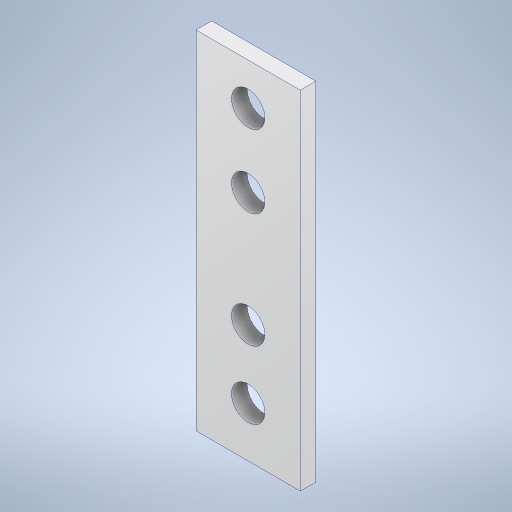
# Autodesk Inventor part: wheel_setter_plate
Saved by Autodesk Inventor 2024.1 (Build 281209000, 209)
## iProperties
Created: 2025-02-03
Part Number: wheel_setter_plate
Material: アルミニウム 6061
Document SubType Name: Sheet Metal
Designer: hibik
Density: 2.7 g/cm^3
Sheet Metal Rule: Default_mm
Appearance: アルミニウム - フラット
Author: hibik
Autodesk Inventor part; units mm, degrees
ref_plane "YZ Plane" through (0, 0, 0) normal (1, 0, 0) x (0, 1, 0)
ref_plane "XZ Plane" through (0, 0, 0) normal (0, 1, 0) x (-1, 0, 0)
ref_plane "XY Plane" through (0, 0, 0) normal (0, 0, 1) x (1, 0, 0)
sketch "スケッチ1" plane through (0, 0, 0) normal (0, 0, 1) x (1, 0, 0)
  line L0 (0, 0) -> (10, 0)
  line L1 (10, 0) -> (10, 35)
  line L2 (10, 35) -> (0, 35)
  line L3 (0, 35) -> (0, 0)
  circle A0 centre (5, 31) radius 1.6
  circle A1 centre (5, 24) radius 1.6
  line L4 (0, 18) -> (10, 18)
  circle A2 centre (5, 13) radius 1.6
  circle A3 centre (5, 6.5) radius 1.6
  line L5 (0, 20) -> (10, 20)
  line L6 (0, 27.5) -> (10, 27.5)
  line L7 (0, 0) -> (10, 0)
  line L8 (10, 0) -> (10, 1.7632)
  line L9 (0, 1.7632) -> (0, 0)
  point P0 (5, 35)
  dimension "d0" = 10
  dimension "d1" = 35
  dimension "d3" = 3.2
  dimension "d4" = 3.2
  dimension "d6" = 7
  dimension "d7" = 18
  dimension "d8" = 3.2
  dimension "d9" = 3.2
  dimension "d10" = 6.5
  dimension "d11" = 5
  dimension "d12" = 15
  measures "d0" distance of L2.end L1.end
  measures "d1" distance of L1.end L0.end
  measures "d3" diameter of A0
  measures "d4" diameter of A1
  measures "d6" distance of A1.centre A0.centre
  measures "d7" distance between parallel lines of L0 L4
  measures "d8" diameter of A2
  measures "d9" diameter of A3
  measures "d10" distance from line of L0 A3.centre
  measures "d11" distance from line of L4 A2.centre
  measures "d12" distance between parallel lines of L2 L5
extrude "プレート1" add sketch "スケッチ1" along normal blind 1.5
sketch "スケッチ2" plane through (0, 0, 1.5) normal (0, 0, 1) x (1, 0, 0)
  line L0 (0, 35) -> (0, 0) projected
  line L1 (10, 0) -> (10, 35) projected
  line L2 (0, 0) -> (10, 0)
  line L3 (10, 0) -> (10, 1.7)
  line L4 (10, 1.7) -> (0, 1.7)
  line L5 (0, 1.7) -> (0, 0)
  dimension "d14" = 1.7
  constraints: 8 end point, 2 parallel, 1 horizontal, 1 perpendicular, 1 point on line
  measures "d14" distance between parallel lines of L2 L4
extrude "切り取り1" cut sketch "スケッチ2" against normal blind 1.5
equation "\"d15\" = Thickness"
equation "\"d2\" = Thickness"
equation "\"BendRadius\" = Thickness"
equation "\"BendReliefWidth\" = Thickness"
equation "\"BendReliefDepth\" = 0.5 * Thickness"
equation "\"CornerReliefSize\" = 4 * Thickness"
equation "\"MinimumRemnant\" = 2 * Thickness"
equation "\"TransitionRadius\" = BendRadius"
equation "\"JacobiRadiusSize\" = BendRadius"
equation "\"GapSize\" = Thickness"
equation "\"Thickness\" = 1.5"
